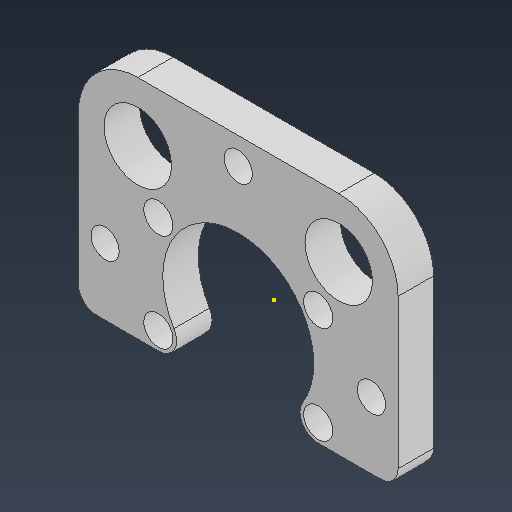
# Autodesk Inventor part: unit-base5
Saved by Autodesk Inventor 2021 (Build 250183000, 183)
## iProperties
Created: 2021-07-14
Part Number: unit-base5
Material: 一般
Document SubType Name: Modeling
Designer: yuta0
Density: 1 g/cm^3
Appearance: 既定
購入先: 印刷
在庫数: 0.0
Author: yuta0
Autodesk Inventor part; units mm, degrees
ref_plane "YZ Plane" through (0, 0, 0) normal (1, 0, 0) x (0, 1, 0)
ref_plane "XZ Plane" through (0, 0, 0) normal (0, 1, 0) x (-1, 0, 0)
ref_plane "XY Plane" through (0, 0, 0) normal (0, 0, 1) x (1, 0, 0)
sketch "スケッチ1" plane through (0, 0, 0) normal (0, 0, 1) x (1, 0, 0)
  line L0 (18, -18) -> (-18, -18)
  line L1 (-18, -18) -> (-18, 18)
  line L2 (-18, 18) -> (18, 18)
  line L3 (18, 18) -> (18, -18)
  line L4 (18, -18) -> (-18, 18) construction
  line L5 (-18, -18) -> (18, 18) construction
  point P0 (0, 0)
  point P1 (0, 0)
  dimension "d34" = 36
  dimension "d35" = 36
  constraints: 12 end point, 2 parallel, 1 coincident, 1 horizontal, 1 midpoint, 1 perpendicular
  measures "d34" distance of L1.end L2.end
  measures "d35" distance of L0.end L1.end
extrude "押し出し1" add sketch "スケッチ1" along normal blind 4
sketch "スケッチ3" plane through (0, 0, 4) normal (0, 0, 1) x (1, 0, 0)
  line L0 (-9, -5.5) -> (9, -5.5)
  line L1 (9, -5.5) -> (9, 5.5)
  line L2 (9, 5.5) -> (-9, 5.5)
  line L3 (-9, 5.5) -> (-9, -5.5)
  line L4 (-9, -5.5) -> (9, 5.5) construction
  line L5 (9, -5.5) -> (-9, 5.5) construction
  point P0 (0, 0)
  dimension "d18" = 18
  dimension "d19" = 11
  constraints: 12 end point, 2 midpoint, 2 parallel, 1 horizontal, 1 perpendicular
  measures "d18" distance of L2.end L1.end
  measures "d19" distance of L1.end L0.end
hole "穴2" at (-9, 5.5, 4) at (-9, -5.5, 4) at (9, -5.5, 4) at (9, 5.5, 4) direction (0, 0, -1) diameter 3.3 end through all
sketch "スケッチ4" plane through (0, 0, 4) normal (0, 0, 1) x (1, 0, 0)
  circle A0 centre (0, 0) radius 8.5
  dimension "d27" = 17
  constraints: 1 centre point, 1 coincident
  measures "d27" diameter of A0
extrude "押し出し2" cut sketch "スケッチ4" against normal through all
sketch "スケッチ5" plane through (0, 0, 4) normal (0, 0, 1) x (1, 0, 0)
  circle A0 centre (0, 0) radius 15
  point P0 (0, 15)
  point P1 (-15, 0)
  point P2 (0, -15)
  point P3 (15, 0)
  dimension "d36" = 30
  dimension "d39" = 360
  constraints: 1 coincident, 1 vertical alignment, 7 other
hole "穴3" at (15, 0, 4) at (-15, 0, 4) at (0, 15, 4) direction (0, 0, -1) diameter 3.2 end through all clearance for "Flat Head Machine Screw" size "M3" standard "Ansi Metric M Profile"
sketch "スケッチ6" plane through (0, 0, 4) normal (0, 0, 1) x (1, 0, 0)
  circle A0 centre (0, 0) radius 16
  point P0 (-11.3137, 11.3137)
  point P1 (-11.3137, -11.3137)
  point P2 (11.3137, -11.3137)
  point P3 (11.3137, 11.3137)
  dimension "d48" = 32
  dimension "d51" = 360
  constraints: 1 coincident, 1 horizontal alignment, 8 other
hole "穴4" at (-11.3137, 11.3137, 4) at (-11.3137, -11.3137, 4) at (11.3137, -11.3137, 4) at (11.3137, 11.3137, 4) direction (0, 0, -1) diameter 4.3 end through all counterbore diameter 7.6 counterbore depth 10 clearance for "Socket Head Cap Screw" size "M4" standard "Ansi Metric M Profile"
sketch "スケッチ9" plane through (0, 0, 4) normal (0, 0, 1) x (1, 0, 0)
  line L0 (-11, -7.5) -> (11, -7.5)
  line L1 (11, -7.5) -> (11, 7.5)
  line L2 (11, 7.5) -> (-11, 7.5)
  line L3 (-11, 7.5) -> (-11, -7.5)
  line L4 (-11, -7.5) -> (11, 7.5) construction
  line L5 (11, -7.5) -> (-11, 7.5) construction
  line L6 (-18, 18) -> (-18, -18) projected
  line L7 (-18, -7.5) -> (18, -7.5)
  line L8 (18, -7.5) -> (18, -18)
  line L9 (18, -18) -> (-18, -18)
  line L10 (-18, -18) -> (-18, -7.5)
  line L11 (18, -18) -> (18, 18) projected
  point P0 (0, 0)
  point P1 (18, -11.3137)
  point P2 (18, 11.3137)
  point P3 (-18, -11.3137)
  dimension "d71" = 22
  dimension "d72" = 15
  constraints: 20 end point, 4 parallel, 3 point on line, 2 horizontal, 2 midpoint, 2 perpendicular
  measures "d71" distance of L2.end L1.end
  measures "d72" distance of L1.end L0.end
extrude "押し出し5" cut sketch "スケッチ9" against normal through all contours L0 L7 L8 L9 L6
fillet "フィレット2" radius 2 4 edges at (-4, -7.5, 2) (4, -7.5, 2) (-18, -7.5, 2) (18, -7.5, 2)
sketch "スケッチ11" plane through (0, 0, 0) normal (0, 0, -1) x (-1, 0, 0)
  point P0 (0, 0)
fillet "フィレット4" radius 6.6865 2 edges at (-18, 18, 2) (18, 18, 2)
